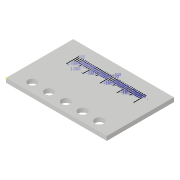
# Autodesk Inventor part: laser test
Saved by Autodesk Inventor 2018 (Build 220112000, 112)
## iProperties
Created: 2019-09-20
Part Number: laser test
Material: Generic
Document SubType Name: Modeling
Designer: ball
Density: 1 g/cm^3
Appearance: Default
Author: ball
Autodesk Inventor part; units mm, degrees
ref_plane "YZ Plane" through (0, 0, 0) normal (1, 0, 0) x (0, 1, 0)
ref_plane "XZ Plane" through (0, 0, 0) normal (0, 1, 0) x (-1, 0, 0)
ref_plane "XY Plane" through (0, 0, 0) normal (0, 0, 1) x (1, 0, 0)
sketch "Sketch1" plane through (0, 0, 0) normal (0, 1, 0) x (-1, 0, 0)
  line L0 (0, 0) -> (-152.4, 0)
  line L1 (-152.4, 0) -> (-152.4, -101.6)
  line L2 (-152.4, -101.6) -> (0, -101.6)
  line L3 (0, -101.6) -> (0, 0)
  circle A0 centre (-25.4, -14.2875) radius 6.35
  circle A1 centre (-50.8, -14.2875) radius 6.4135
  circle A2 centre (-76.2, -14.2875) radius 6.477
  circle A3 centre (-101.6, -14.2875) radius 6.604
  circle A4 centre (-127, -14.2875) radius 6.731
  line L4 (-22.178, -1.7823) -> (-15.0248, -1.7823) construction
  line L5 (-15.0248, -1.7823) -> (-15.0248, -4.5598) construction
  line L6 (-15.0248, -4.5598) -> (-22.178, -4.5598) construction
  line L7 (-22.178, -4.5598) -> (-22.178, -1.7823) construction
  line L8 (-49.534, -2.7734) -> (-41.4027, -2.7734) construction
  line L9 (-41.4027, -2.7734) -> (-41.4027, -4.3616) construction
  line L10 (-41.4027, -4.3616) -> (-49.534, -4.3616) construction
  line L11 (-49.534, -4.3616) -> (-49.534, -2.7734) construction
  line L12 (-76.4936, -2.1788) -> (-70.6496, -2.1788) construction
  line L13 (-70.6496, -2.1788) -> (-70.6496, -8.2743) construction
  line L14 (-70.6496, -8.2743) -> (-76.4936, -8.2743) construction
  line L15 (-76.4936, -8.2743) -> (-76.4936, -2.1788) construction
  line L16 (-99.6868, -2.377) -> (-93.8428, -2.377) construction
  line L17 (-93.8428, -2.377) -> (-93.8428, -5.5534) construction
  line L18 (-93.8428, -5.5534) -> (-99.6868, -5.5534) construction
  line L19 (-99.6868, -5.5534) -> (-99.6868, -2.377) construction
  line L20 (-126.4482, -3.1699) -> (-120.6041, -3.1699) construction
  line L21 (-120.6041, -3.1699) -> (-120.6041, -6.3464) construction
  line L22 (-120.6041, -6.3464) -> (-126.4482, -6.3464) construction
  line L23 (-126.4482, -6.3464) -> (-126.4482, -3.1699) construction
  circle A5 centre (98.0568, -52.9534) radius 11.3595
  line L24 (110.7568, -52.9534) -> (105.4477, -74.5496) construction
  line L25 (105.4477, -74.5496) -> (102.5257, -83.1159) construction
  line L26 (102.5257, -83.1159) -> (85.1766, -74.5496) construction
  spline S0 degree 3 poles (110.7568, -52.9534) (105.4477, -74.5496) (102.5257, -83.1159) (85.1766, -74.5496) knots 1 1 1 1 2 2 2 2
  line L27 (-12.1084, -90.1112) -> (-75.5229, -90.1112)
  line L28 (-12.1084, -90.1112) -> (-12.1084, -63.1237)
  line L29 (-14.6484, -90.1112) -> (-14.6484, -78.9358)
  line L30 (-17.1884, -90.1112) -> (-17.1884, -78.9358)
  line L31 (-19.7284, -90.1112) -> (-19.7284, -78.9358)
  line L32 (-22.2684, -90.1112) -> (-22.2684, -78.9358)
  line L33 (-24.8084, -90.1112) -> (-24.8084, -74.2362)
  line L34 (-29.429, -90.1112) -> (-29.429, -78.9358)
  dimension "d0" = 152.4
  dimension "d1" = 101.6
  dimension "d2" = 12.7
  dimension "d3" = 12.827
  dimension "d4" = 12.954
  dimension "d5" = 13.208
  dimension "d6" = 13.462
  dimension "d7" = 25.4
  dimension "d8" = 25.4
  dimension "d9" = 25.4
  dimension "d10" = 25.4
  dimension "d11" = 25.4
  dimension "d12" = 25.4
  dimension "d14" = 2.54
  dimension "d15" = 2.54
  dimension "d16" = 2.54
  dimension "d17" = 2.54
  dimension "d18" = 2.54
  constraints: 24 end point, 6 centre point, 6 point on line, 5 vertical, 3 perpendicular, 2 horizontal, 2 parallel, 13 other
  measures "d0" distance of L2.end L1.end
  measures "d1" distance of L1.end L0.end
  measures "d2" diameter of A0
  measures "d3" diameter of A1
  measures "d4" diameter of A2
  measures "d5" diameter of A3
  measures "d6" diameter of A4
  measures "d7" distance of A1.centre A0.centre
  measures "d8" distance of A2.centre A1.centre
  measures "d9" distance of A3.centre A2.centre
  measures "d10" distance of A4.centre A3.centre
  measures "d11" distance from line of L1 A4.centre
  measures "d12" distance from line of L3 A0.centre
  measures "d14" distance between parallel lines of L28 L29
  measures "d15" distance between parallel lines of L29 L30
  measures "d16" distance between parallel lines of L30 L31
  measures "d17" distance between parallel lines of L32 L31
  measures "d18" distance between parallel lines of L32 L33
extrude "Extrusion1" add sketch "Sketch1" along normal blind 6.35 contours L3 L2 L1 L0
sketch "Sketch2" plane through (0, 6.35, 0) normal (0, 1, 0) x (1, 0, 0)
  line L0 (54.8132, 82.9766) -> (54.8132, 74.0866)
  line L1 (57.3532, 82.9766) -> (57.3532, 74.0866)
  line L2 (59.8932, 82.9766) -> (59.8932, 74.0866)
  line L3 (62.4332, 82.9766) -> (62.4332, 74.0866)
  line L4 (64.9732, 82.9766) -> (64.9732, 70.2766)
  line L5 (67.5132, 82.9766) -> (67.5132, 74.0866)
  line L6 (70.0532, 82.9766) -> (70.0532, 74.0866)
  line L7 (72.5932, 82.9766) -> (72.5932, 74.0866)
  line L8 (75.1332, 82.9766) -> (75.1332, 74.0866)
  line L9 (77.6732, 82.9766) -> (77.6732, 63.9266)
  line L10 (29.4132, 82.713) -> (29.4132, 73.823)
  line L11 (31.9532, 82.713) -> (31.9532, 73.823)
  line L12 (34.4932, 82.713) -> (34.4932, 73.823)
  line L13 (37.0332, 82.713) -> (37.0332, 73.823)
  line L14 (39.5732, 82.713) -> (39.5732, 70.013)
  line L15 (42.1132, 82.713) -> (42.1132, 73.823)
  line L16 (44.6532, 82.713) -> (44.6532, 73.823)
  line L17 (47.1932, 82.713) -> (47.1932, 73.823)
  line L18 (49.7332, 82.713) -> (49.7332, 73.823)
  line L19 (52.2732, 82.713) -> (52.2732, 63.663)
  line L20 (26.8732, 82.713) -> (26.8732, 63.663)
  line L21 (80.2132, 82.87) -> (80.2132, 73.98)
  line L22 (82.7532, 82.87) -> (82.7532, 73.98)
  line L23 (85.2932, 82.87) -> (85.2932, 73.98)
  line L24 (87.8332, 82.87) -> (87.8332, 73.98)
  line L25 (90.3732, 82.87) -> (90.3732, 70.17)
  line L26 (92.9132, 82.87) -> (92.9132, 73.98)
  line L27 (95.4532, 82.87) -> (95.4532, 73.98)
  line L28 (97.9932, 82.87) -> (97.9932, 73.98)
  line L29 (100.5332, 82.87) -> (100.5332, 73.98)
  line L30 (103.0732, 82.87) -> (103.0732, 63.82)
  line L31 (105.6132, 83.1064) -> (105.6132, 74.2164)
  line L32 (108.1532, 83.1064) -> (108.1532, 74.2164)
  line L33 (110.6932, 83.1064) -> (110.6932, 74.2164)
  line L34 (113.2332, 83.1064) -> (113.2332, 74.2164)
  line L35 (115.7732, 83.1064) -> (115.7732, 70.4064)
  line L36 (118.3132, 83.1064) -> (118.3132, 74.2164)
  line L37 (120.8532, 83.1064) -> (120.8532, 74.2164)
  line L38 (123.3932, 83.1064) -> (123.3932, 74.2164)
  line L39 (125.9332, 83.1064) -> (125.9332, 74.2164)
  line L40 (128.4732, 83.1064) -> (128.4732, 64.0564)
  point P0 (0, 0)
  dimension "d22" = 8.89
  dimension "d24" = 2.54
  dimension "d25" = 2.54
  dimension "d26" = 2.54
  dimension "d27" = 2.54
  dimension "d28" = 2.54
  dimension "d29" = 2.54
  dimension "d30" = 2.54
  dimension "d31" = 2.54
  dimension "d33" = 2.54
  dimension "d34" = 8.89
  dimension "d35" = 2.54
  dimension "d36" = 2.54
  dimension "d37" = 2.54
  dimension "d38" = 2.54
  dimension "d39" = 2.54
  dimension "d40" = 2.54
  dimension "d41" = 2.54
  dimension "d42" = 2.54
  dimension "d43" = 2.54
  dimension "d44" = 25.4
  dimension "d45" = 2.54
  dimension "d46" = 8.89
  dimension "d47" = 2.54
  dimension "d48" = 2.54
  dimension "d49" = 2.54
  dimension "d50" = 2.54
  dimension "d51" = 2.54
  dimension "d52" = 2.54
  dimension "d53" = 2.54
  dimension "d54" = 2.54
  dimension "d55" = 2.54
  dimension "d56" = 2.54
  dimension "d57" = 8.89
  dimension "d58" = 2.54
  dimension "d59" = 2.54
  dimension "d60" = 2.54
  dimension "d61" = 2.54
  dimension "d62" = 2.54
  dimension "d63" = 2.54
  dimension "d64" = 2.54
  dimension "d65" = 2.54
  dimension "d66" = 2.54
  dimension "d67" = 2.54
  constraints: 82 end point, 41 vertical
  measures "d22" distance of L0.start L0.end
  measures "d24" distance between parallel lines of L1 L0
  measures "d25" distance between parallel lines of L2 L1
  measures "d26" distance between parallel lines of L2 L3
  measures "d27" distance between parallel lines of L4 L5
  measures "d28" distance between parallel lines of L4 L3
  measures "d29" distance between parallel lines of L5 L6
  measures "d30" distance between parallel lines of L6 L7
  measures "d31" distance between parallel lines of L7 L8
  measures "d33" distance between parallel lines of L8 L9
  measures "d34" distance of L10.start L10.end
  measures "d35" distance between parallel lines of L11 L10
  measures "d36" distance between parallel lines of L12 L11
  measures "d37" distance between parallel lines of L12 L13
  measures "d38" distance between parallel lines of L14 L15
  measures "d39" distance between parallel lines of L14 L13
  measures "d40" distance between parallel lines of L15 L16
  measures "d41" distance between parallel lines of L16 L17
  measures "d42" distance between parallel lines of L17 L18
  measures "d43" distance between parallel lines of L18 L19
  measures "d44" distance between parallel lines of L20 L19
  measures "d45" distance between parallel lines of L19 L0
  measures "d46" distance of L21.start L21.end
  measures "d47" distance between parallel lines of L22 L21
  measures "d48" distance between parallel lines of L23 L22
  measures "d49" distance between parallel lines of L23 L24
  measures "d50" distance between parallel lines of L25 L26
  measures "d51" distance between parallel lines of L25 L24
  measures "d52" distance between parallel lines of L26 L27
  measures "d53" distance between parallel lines of L27 L28
  measures "d54" distance between parallel lines of L28 L29
  measures "d55" distance between parallel lines of L29 L30
  measures "d56" distance between parallel lines of L9 L21
  measures "d57" distance of L31.start L31.end
  measures "d58" distance between parallel lines of L32 L31
  measures "d59" distance between parallel lines of L33 L32
  measures "d60" distance between parallel lines of L33 L34
  measures "d61" distance between parallel lines of L35 L36
  measures "d62" distance between parallel lines of L35 L34
  measures "d63" distance between parallel lines of L36 L37
  measures "d64" distance between parallel lines of L37 L38
  measures "d65" distance between parallel lines of L38 L39
  measures "d66" distance between parallel lines of L39 L40
  measures "d67" distance between parallel lines of L30 L31
body "Solid1"
